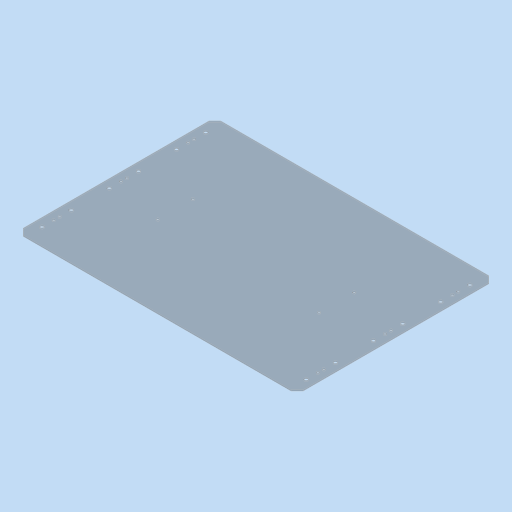
# Autodesk Inventor part: enc-SidePanel 500x708
Saved by Autodesk Inventor 2023.2 (Build 272271000, 271)
## iProperties
Created: 2023-11-30
Part Number: enc-SidePanel 500x708
Material: Generisch
Document SubType Name: Modeling
Designer: Nils Bade
Density: 1 g/cm^3
Appearance: PVC Verglasung
Author: Nils Bade
Autodesk Inventor part; units mm, degrees
ref_plane "YZ Plane" through (0, 0, 0) normal (1, 0, 0) x (0, 1, 0)
ref_plane "XZ Plane" through (0, 0, 0) normal (0, 1, 0) x (-1, 0, 0)
ref_plane "XY Plane" through (0, 0, 0) normal (0, 0, 1) x (1, 0, 0)
sketch "Skizze1" plane through (0, 0, 0) normal (0, 1, 0) x (-1, 0, 0)
  line L0 (0, 0) -> (-708, 0)
  line L1 (-708, 0) -> (-708, 500)
  line L2 (-708, 500) -> (0, 500)
  line L3 (0, 500) -> (0, 0)
  line L4 (-354, 0) -> (-354, 500) construction
  line L5 (0, 250) -> (-708, 250) construction
  line L6 (-150, 0) -> (-150, 500) construction
  line L7 (-558, 0) -> (-558, 500) construction
  line L8 (-708, 420) -> (0, 420) construction
  line L9 (0, 80) -> (-708, 80) construction
  line L10 (-688, 480) -> (-688, 20) construction
  line L11 (-688, 20) -> (-20, 20) construction
  line L12 (-20, 20) -> (-20, 480) construction
  line L13 (-20, 480) -> (-688, 480) construction
  line L14 (-28, 372.5) -> (-12, 372.5) construction
  line L15 (-12, 372.5) -> (-12, 467.5) construction
  line L16 (-12, 467.5) -> (-28, 467.5) construction
  line L17 (-28, 467.5) -> (-28, 372.5) construction
  line L18 (-28, 372.5) -> (-12, 467.5) construction
  line L19 (-12, 372.5) -> (-28, 467.5) construction
  line L20 (-102.5, 488) -> (-197.5, 488) construction
  line L21 (-197.5, 488) -> (-197.5, 472) construction
  line L22 (-197.5, 472) -> (-102.5, 472) construction
  line L23 (-102.5, 472) -> (-102.5, 488) construction
  line L24 (-102.5, 488) -> (-197.5, 472) construction
  line L25 (-197.5, 488) -> (-102.5, 472) construction
  line L26 (-306.5, 488) -> (-401.5, 488) construction
  line L27 (-401.5, 488) -> (-401.5, 472) construction
  line L28 (-401.5, 472) -> (-306.5, 472) construction
  line L29 (-306.5, 472) -> (-306.5, 488) construction
  line L30 (-306.5, 488) -> (-401.5, 472) construction
  line L31 (-401.5, 488) -> (-306.5, 472) construction
  circle A0 centre (-20, 412.5) radius 3.25
  circle A1 centre (-20, 383) radius 4.5
  circle A2 centre (-20, 427.5) radius 3.25
  circle A3 centre (-20, 457) radius 4.5
  circle A4 centre (-142.5, 480) radius 3.25
  circle A5 centre (-113, 480) radius 4.5
  circle A6 centre (-317, 480) radius 4.5
  circle A7 centre (-346.5, 480) radius 3.25
  circle A8 centre (-157.5, 480) radius 3.25
  circle A9 centre (-187, 480) radius 4.5
  circle A10 centre (-391, 480) radius 4.5
  circle A11 centre (-361.5, 480) radius 3.25
  circle A12 centre (-688, 412.5) radius 3.25
  circle A13 centre (-688, 383) radius 4.5
  circle A14 centre (-688, 457) radius 4.5
  circle A15 centre (-688, 427.5) radius 3.25
  circle A16 centre (-565.5, 480) radius 3.25
  circle A17 centre (-595, 480) radius 4.5
  circle A18 centre (-550.5, 480) radius 3.25
  circle A19 centre (-521, 480) radius 4.5
  circle A20 centre (-20, 43) radius 4.5
  circle A21 centre (-20, 72.5) radius 3.25
  circle A22 centre (-150, 205.5) radius 3.25
  line L32 (-138.5, 196) -> (-161.5, 196) construction
  line L33 (-161.5, 196) -> (-161.5, 304) construction
  line L34 (-161.5, 304) -> (-138.5, 304) construction
  line L35 (-138.5, 304) -> (-138.5, 196) construction
  line L36 (-138.5, 196) -> (-161.5, 304) construction
  line L37 (-161.5, 196) -> (-138.5, 304) construction
  circle A23 centre (-150, 294.5) radius 3.25
  circle A24 centre (-558, 205.5) radius 3.25
  circle A25 centre (-558, 294.5) radius 3.25
  circle A26 centre (-20, 117) radius 4.5
  circle A27 centre (-20, 87.5) radius 3.25
  circle A28 centre (-688, 43) radius 4.5
  circle A29 centre (-688, 72.5) radius 3.25
  circle A30 centre (-688, 87.5) radius 3.25
  circle A31 centre (-688, 117) radius 4.5
  circle A32 centre (-20, 213) radius 4.5
  circle A33 centre (-20, 242.5) radius 3.25
  circle A34 centre (-20, 257.5) radius 3.25
  circle A35 centre (-20, 287) radius 4.5
  circle A36 centre (-688, 242.5) radius 3.25
  circle A37 centre (-688, 213) radius 4.5
  circle A38 centre (-688, 287) radius 4.5
  circle A39 centre (-688, 257.5) radius 3.25
  point P0 (-20, 420)
  point P1 (-150, 480)
  point P2 (-354, 480)
  point P3 (-150, 250)
  dimension "d0" = 708
  dimension "d1" = 500
  dimension "d2" = 80
  dimension "d3" = 80
  dimension "d4" = 150
  dimension "d5" = 150
  dimension "d6" = 20
  dimension "d7" = 16
  dimension "d8" = 95
  dimension "d9" = 95
  dimension "d10" = 16
  dimension "d11" = 95
  dimension "d12" = 16
  dimension "d13" = 6.5
  dimension "d14" = 7.5
  dimension "d15" = 9
  dimension "d16" = 37
  dimension "d17" = 6.5
  dimension "d18" = 9
  dimension "d19" = 7.5
  dimension "d20" = 37
  dimension "d21" = 6.5
  dimension "d22" = 9
  dimension "d23" = 7.5
  dimension "d24" = 37
  dimension "d30" = 6.5
  dimension "d31" = 44.5
  dimension "d32" = 23
  dimension "d33" = 108
  dimension "d34" = 6.5
  dimension "d35" = 9
  dimension "d36" = 7.5
  dimension "d37" = 37
  dimension "d38" = 6.5
  dimension "d39" = 9
  dimension "d42" = 7.5
  dimension "d43" = 37
  constraints: 76 end point, 40 centre point, 29 symmetric about line, 21 point on line, 14 midpoint, 12 parallel, 10 perpendicular, 5 horizontal, 32 other
  measures "d0" distance of L0.start L0.end
  measures "d1" distance of L2.end L0.start
  measures "d2" distance between parallel lines of L2 L8
  measures "d3" distance between parallel lines of L0 L9
  measures "d4" distance between parallel lines of L3 L6
  measures "d5" distance between parallel lines of L1 L7
  measures "d6" distance between parallel lines of L1 L10
  measures "d7" distance of L16.end L15.end
  measures "d8" distance of L15.end L14.end
  measures "d9" distance of L22.end L21.end
  measures "d10" distance of L21.end L20.end
  measures "d11" distance of L28.end L27.end
  measures "d12" distance of L27.end L26.end
  measures "d13" diameter of A0
  measures "d14" distance from line of L8 A0.centre
  measures "d15" diameter of A1
  measures "d16" distance from line of L8 A1.centre
  measures "d17" diameter of A4
  measures "d18" diameter of A5
  measures "d19" distance from line of L6 A4.centre
  measures "d20" distance from line of L6 A5.centre
  measures "d21" diameter of A7
  measures "d22" diameter of A6
  measures "d23" distance from line of L4 A7.centre
  measures "d24" distance from line of L4 A6.centre
  measures "d30" diameter of A22
  measures "d31" distance from line of L5 A22.centre
  measures "d32" distance of L33.end L34.end
  measures "d33" distance of L32.end L33.end
  measures "d34" diameter of A21
  measures "d35" diameter of A20
  measures "d36" distance from line of L9 A21.centre
  measures "d37" distance from line of L9 A20.centre
  measures "d38" diameter of A33
  measures "d39" diameter of A32
  measures "d42" distance from line of L5 A33.centre
  measures "d43" distance from line of L5 A32.centre
extrude "Extrusion1" add sketch "Skizze1" along normal blind 3 contours L0 L1 L2 L3 | A4 | A5 | A6 | A7 | A8 | A9 | A10 | A11 | A16 | A17 | A18 | A19
chamfer "Fase1" distance 15 angle 45 4 edges at (0, 1.5, 500) (708, 1.5, 500) (708, 1.5, 0) (0, 1.5, 0)
equation "\"d5\" = d4"
equation "\"d17\" = d13"
equation "\"d18\" = d15"
equation "\"d19\" = d14"
equation "\"d20\" = d16"
equation "\"d21\" = d13"
equation "\"d22\" = d15"
equation "\"d23\" = d14"
equation "\"d24\" = d16"
equation "\"d34\" = d13"
equation "\"d35\" = d15"
equation "\"d36\" = d14"
equation "\"d37\" = d16"
equation "\"d38\" = d13"
equation "\"d39\" = d15"
equation "\"d42\" = d14"
equation "\"d43\" = d16"
